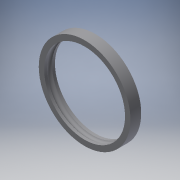
# Autodesk Inventor part: outer ring
Saved by Autodesk Inventor 2017 (Build 210142000, 142)
## iProperties
Created: 2017-12-09
Part Number: outer ring
Material: Generic
Document SubType Name: Modeling
Designer: prakhar
Density: 1 g/cm^3
Appearance: Default
Author: prakhar
Autodesk Inventor part; units mm, degrees
ref_plane "YZ Plane" through (0, 0, 0) normal (1, 0, 0) x (0, 1, 0)
ref_plane "XZ Plane" through (0, 0, 0) normal (0, 1, 0) x (-1, 0, 0)
ref_plane "XY Plane" through (0, 0, 0) normal (0, 0, 1) x (1, 0, 0)
sketch "Sketch1" plane through (0, 0, 0) normal (0, 1, 0) x (-1, 0, 0)
  line L0 (50.7746, 6.35) -> (47.625, 6.35)
  line L1 (47.625, 6.35) -> (47.625, -6.35)
  line L2 (47.625, -6.35) -> (50.7746, -6.35)
  line L3 (50.7746, -6.35) -> (50.7746, 6.35)
  arc A0 (47.625, -2.9696) -> (47.625, 2.9696) centre (45.9105, 0) ccw
  line L4 (0, -8.89) -> (0, 8.89) projected
  point P0 (0, 0)
  point P1 (50.7746, 0)
  dimension "d1" = 47.625
  dimension "d2" = 3.1496
  dimension "d3" = 6.35
  dimension "d4" = 6.35
  dimension "d5" = 1.7145
  dimension "d6" = 3.429
  constraints: 8 end point, 2 parallel, 2 point on circle, 2 point on line, 1 centre point, 1 horizontal, 1 horizontal alignment, 1 midpoint, 1 perpendicular
  measures "d1" distance from line of point (0, 0) L1
  measures "d2" distance of L1.end L2.end
  measures "d3" distance from line of L2 point (0, 0)
  measures "d4" distance from line of point (0, 0) L0
  measures "d5" distance centre to line of A0 L1
  measures "d6" radius of A0
revolve "Revolution1" add sketch "Sketch1" angle 360 about axis through (0, 0, -10) along (0, 0, 1) contours L3 L2 L1 A0 L0
body "Solid1"
